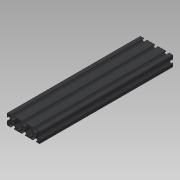
# Autodesk Inventor part: 1030
Saved by Autodesk Inventor 2013 (Build 170138000, 138)
## iProperties
Company: 80/20 Inc.
Created: 2013-09-06
Part Number: 1030
Material: Generic
Document SubType Name: Modeling
Density: 1 g/cm^3
Catalog Web Link: 8020.net
Vendor: 80/20 Inc.
Engineer: Ross Bowman
Author: Ross Bowman
Keywords: T-Slot, Extrusion, 80/20, 8020, Quick Frame, HT
Autodesk Inventor part; units mm, degrees
ref_plane "YZ Plane" through (0, 0, 0) normal (1, 0, 0) x (0, 1, 0)
ref_plane "XZ Plane" through (0, 0, 0) normal (0, 1, 0) x (-1, 0, 0)
ref_plane "XY Plane" through (0, 0, 0) normal (0, 0, 1) x (1, 0, 0)
sketch "Sketch1" plane through (0, 0, 0) normal (0, 0, 1) x (1, 0, 0)
  circle A0 centre (25.4, 0) radius 2.6035
  circle A1 centre (0, 0) radius 2.6035
  circle A2 centre (-25.4, 0) radius 2.6035
  arc A3 (19.9657, -3.8718) -> (20.8956, -1.6267) centre (17.7206, -1.6267) ccw
  line L0 (14.2657, -9.5718) -> (19.9657, -3.8718)
  arc A4 (13.1521, -10.033) -> (14.2657, -9.5718) centre (13.1521, -8.4582) ccw
  line L1 (12.2479, -10.033) -> (13.1521, -10.033)
  arc A5 (11.1343, -9.5718) -> (12.2479, -10.033) centre (12.2479, -8.4582) ccw
  line L2 (5.4343, -3.8717) -> (11.1343, -9.5718)
  arc A6 (4.5044, -1.6267) -> (5.4343, -3.8717) centre (7.6794, -1.6267) ccw
  line L3 (4.5044, 1.6267) -> (4.5044, -1.6267)
  arc A7 (5.4343, 3.8717) -> (4.5044, 1.6267) centre (7.6794, 1.6267) ccw
  line L4 (11.1343, 9.5718) -> (5.4343, 3.8717)
  arc A8 (12.2479, 10.033) -> (11.1343, 9.5718) centre (12.2479, 8.4582) ccw
  line L5 (13.1521, 10.033) -> (12.2479, 10.033)
  arc A9 (14.2657, 9.5718) -> (13.1521, 10.033) centre (13.1521, 8.4582) ccw
  line L6 (19.9657, 3.8717) -> (14.2657, 9.5718)
  arc A10 (20.8956, 1.6267) -> (19.9657, 3.8717) centre (17.7206, 1.6267) ccw
  line L7 (20.8956, -1.6267) -> (20.8956, 1.6267)
  arc A11 (-20.8956, -1.6267) -> (-19.9657, -3.8717) centre (-17.7206, -1.6267) ccw
  line L8 (-20.8956, 1.6267) -> (-20.8956, -1.6267)
  arc A12 (-19.9657, 3.8717) -> (-20.8956, 1.6267) centre (-17.7206, 1.6267) ccw
  line L9 (-14.2657, 9.5718) -> (-19.9657, 3.8717)
  arc A13 (-13.1521, 10.033) -> (-14.2657, 9.5718) centre (-13.1521, 8.4582) ccw
  line L10 (-12.2479, 10.033) -> (-13.1521, 10.033)
  arc A14 (-11.1343, 9.5718) -> (-12.2479, 10.033) centre (-12.2479, 8.4582) ccw
  line L11 (-5.4343, 3.8717) -> (-11.1343, 9.5718)
  arc A15 (-4.5044, 1.6267) -> (-5.4343, 3.8717) centre (-7.6794, 1.6267) ccw
  line L12 (-4.5044, -1.6267) -> (-4.5044, 1.6267)
  arc A16 (-5.4343, -3.8718) -> (-4.5044, -1.6267) centre (-7.6794, -1.6267) ccw
  line L13 (-11.1343, -9.5718) -> (-5.4343, -3.8718)
  arc A17 (-12.2479, -10.033) -> (-11.1343, -9.5718) centre (-12.2479, -8.4582) ccw
  line L14 (-13.1521, -10.033) -> (-12.2479, -10.033)
  arc A18 (-14.2657, -9.5718) -> (-13.1521, -10.033) centre (-13.1521, -8.4582) ccw
  line L15 (-19.9657, -3.8717) -> (-14.2657, -9.5718)
  arc A19 (-1.6267, -4.5044) -> (-3.8717, -5.4343) centre (-1.6267, -7.6794) ccw
  line L16 (-1.6267, -4.5044) -> (1.6267, -4.5044)
  arc A20 (3.8717, -5.4343) -> (1.6267, -4.5044) centre (1.6267, -7.6794) ccw
  line L17 (3.8717, -5.4343) -> (7.1932, -8.7558)
  arc A21 (6.4748, -10.4902) -> (7.1932, -8.7558) centre (6.4748, -9.4742) ccw
  line L18 (6.4748, -10.4902) -> (4.3561, -10.4902)
  arc A22 (4.3561, -10.4902) -> (4.3561, -12.7) centre (4.3561, -11.5951) ccw
  line L19 (4.3561, -12.7) -> (5.3086, -12.7)
  arc A23 (6.3246, -12.7) -> (5.3086, -12.7) centre (5.8166, -12.7) ccw
  line L20 (6.3246, -12.7) -> (9.5504, -12.7)
  arc A24 (10.5664, -12.7) -> (9.5504, -12.7) centre (10.0584, -12.7) ccw
  line L21 (10.5664, -12.7) -> (14.8336, -12.7)
  arc A25 (15.8496, -12.7) -> (14.8336, -12.7) centre (15.3416, -12.7) ccw
  line L22 (15.8496, -12.7) -> (19.0754, -12.7)
  arc A26 (20.0914, -12.7) -> (19.0754, -12.7) centre (19.5834, -12.7) ccw
  line L23 (20.0914, -12.7) -> (21.0439, -12.7)
  arc A27 (21.0439, -12.7) -> (21.0439, -10.4902) centre (21.0439, -11.5951) ccw
  line L24 (21.0439, -10.4902) -> (18.9252, -10.4902)
  arc A28 (18.2068, -8.7558) -> (18.9252, -10.4902) centre (18.9252, -9.4742) ccw
  line L25 (18.2068, -8.7558) -> (21.5283, -5.4343)
  arc A29 (23.7733, -4.5044) -> (21.5283, -5.4343) centre (23.7733, -7.6794) ccw
  line L26 (23.7733, -4.5044) -> (27.0267, -4.5044)
  arc A30 (29.2718, -5.4343) -> (27.0267, -4.5044) centre (27.0267, -7.6794) ccw
  line L27 (29.2718, -5.4343) -> (32.5932, -8.7558)
  arc A31 (31.8748, -10.4902) -> (32.5932, -8.7558) centre (31.8748, -9.4742) ccw
  line L28 (31.8748, -10.4902) -> (29.7561, -10.4902)
  arc A32 (29.7561, -10.4902) -> (29.7561, -12.7) centre (29.7561, -11.5951) ccw
  line L29 (29.7561, -12.7) -> (30.7086, -12.7)
  arc A33 (31.7246, -12.7) -> (30.7086, -12.7) centre (31.2166, -12.7) ccw
  line L30 (31.7246, -12.7) -> (34.9504, -12.7)
  arc A34 (35.9664, -12.7) -> (34.9504, -12.7) centre (35.4584, -12.7) ccw
  line L31 (35.9664, -12.7) -> (35.9918, -12.7)
  arc A35 (35.9918, -12.7) -> (38.1, -10.5918) centre (35.9918, -10.5918) ccw
  line L32 (38.1, -10.5918) -> (38.1, -10.5664)
  arc A36 (38.1, -9.5504) -> (38.1, -10.5664) centre (38.1, -10.0584) ccw
  line L33 (38.1, -9.5504) -> (38.1, -6.3246)
  arc A37 (38.1, -5.3086) -> (38.1, -6.3246) centre (38.1, -5.8166) ccw
  line L34 (38.1, -5.3086) -> (38.1, -4.3561)
  arc A38 (38.1, -4.3561) -> (35.8902, -4.3561) centre (36.9951, -4.3561) ccw
  line L35 (35.8902, -4.3561) -> (35.8902, -6.4748)
  arc A39 (34.1558, -7.1932) -> (35.8902, -6.4748) centre (34.8742, -6.4748) ccw
  line L36 (34.1558, -7.1932) -> (30.8343, -3.8717)
  arc A40 (29.9044, -1.6267) -> (30.8343, -3.8717) centre (33.0794, -1.6267) ccw
  line L37 (29.9044, -1.6267) -> (29.9044, 1.6267)
  arc A41 (30.8343, 3.8718) -> (29.9044, 1.6267) centre (33.0794, 1.6267) ccw
  line L38 (30.8343, 3.8718) -> (34.1558, 7.1932)
  arc A42 (35.8902, 6.4748) -> (34.1558, 7.1932) centre (34.8742, 6.4748) ccw
  line L39 (35.8902, 6.4748) -> (35.8902, 4.3561)
  arc A43 (35.8902, 4.3561) -> (38.1, 4.3561) centre (36.9951, 4.3561) ccw
  line L40 (38.1, 4.3561) -> (38.1, 5.3086)
  arc A44 (38.1, 6.3246) -> (38.1, 5.3086) centre (38.1, 5.8166) ccw
  line L41 (38.1, 6.3246) -> (38.1, 9.5504)
  arc A45 (38.1, 10.5664) -> (38.1, 9.5504) centre (38.1, 10.0584) ccw
  line L42 (38.1, 10.5664) -> (38.1, 10.5918)
  arc A46 (38.1, 10.5918) -> (35.9918, 12.7) centre (35.9918, 10.5918) ccw
  line L43 (35.9918, 12.7) -> (35.9664, 12.7)
  arc A47 (34.9504, 12.7) -> (35.9664, 12.7) centre (35.4584, 12.7) ccw
  line L44 (34.9504, 12.7) -> (31.7246, 12.7)
  arc A48 (30.7086, 12.7) -> (31.7246, 12.7) centre (31.2166, 12.7) ccw
  line L45 (30.7086, 12.7) -> (29.7561, 12.7)
  arc A49 (29.7561, 12.7) -> (29.7561, 10.4902) centre (29.7561, 11.5951) ccw
  line L46 (29.7561, 10.4902) -> (31.8748, 10.4902)
  arc A50 (32.5932, 8.7558) -> (31.8748, 10.4902) centre (31.8748, 9.4742) ccw
  line L47 (32.5932, 8.7558) -> (29.2717, 5.4343)
  arc A51 (27.0267, 4.5044) -> (29.2717, 5.4343) centre (27.0267, 7.6794) ccw
  line L48 (27.0267, 4.5044) -> (23.7733, 4.5044)
  arc A52 (21.5283, 5.4343) -> (23.7733, 4.5044) centre (23.7733, 7.6794) ccw
  line L49 (21.5283, 5.4343) -> (18.2068, 8.7558)
  arc A53 (18.9252, 10.4902) -> (18.2068, 8.7558) centre (18.9252, 9.4742) ccw
  line L50 (18.9252, 10.4902) -> (21.0439, 10.4902)
  arc A54 (21.0439, 10.4902) -> (21.0439, 12.7) centre (21.0439, 11.5951) ccw
  line L51 (21.0439, 12.7) -> (20.0914, 12.7)
  arc A55 (19.0754, 12.7) -> (20.0914, 12.7) centre (19.5834, 12.7) ccw
  line L52 (19.0754, 12.7) -> (15.8496, 12.7)
  arc A56 (14.8336, 12.7) -> (15.8496, 12.7) centre (15.3416, 12.7) ccw
  line L53 (14.8336, 12.7) -> (10.5664, 12.7)
  arc A57 (9.5504, 12.7) -> (10.5664, 12.7) centre (10.0584, 12.7) ccw
  line L54 (9.5504, 12.7) -> (6.3246, 12.7)
  arc A58 (5.3086, 12.7) -> (6.3246, 12.7) centre (5.8166, 12.7) ccw
  line L55 (5.3086, 12.7) -> (4.3561, 12.7)
  arc A59 (4.3561, 12.7) -> (4.3561, 10.4902) centre (4.3561, 11.5951) ccw
  line L56 (4.3561, 10.4902) -> (6.4748, 10.4902)
  arc A60 (7.1932, 8.7558) -> (6.4748, 10.4902) centre (6.4748, 9.4742) ccw
  line L57 (7.1932, 8.7558) -> (3.8717, 5.4343)
  arc A61 (1.6267, 4.5044) -> (3.8717, 5.4343) centre (1.6267, 7.6794) ccw
  line L58 (1.6267, 4.5044) -> (-1.6267, 4.5044)
  arc A62 (-3.8717, 5.4343) -> (-1.6267, 4.5044) centre (-1.6267, 7.6794) ccw
  line L59 (-3.8717, 5.4343) -> (-7.1932, 8.7558)
  arc A63 (-6.4748, 10.4902) -> (-7.1932, 8.7558) centre (-6.4748, 9.4742) ccw
  line L60 (-6.4748, 10.4902) -> (-4.3561, 10.4902)
  arc A64 (-4.3561, 10.4902) -> (-4.3561, 12.7) centre (-4.3561, 11.5951) ccw
  line L61 (-4.3561, 12.7) -> (-5.3086, 12.7)
  arc A65 (-6.3246, 12.7) -> (-5.3086, 12.7) centre (-5.8166, 12.7) ccw
  line L62 (-6.3246, 12.7) -> (-9.5504, 12.7)
  arc A66 (-10.5664, 12.7) -> (-9.5504, 12.7) centre (-10.0584, 12.7) ccw
  line L63 (-10.5664, 12.7) -> (-14.8336, 12.7)
  arc A67 (-15.8496, 12.7) -> (-14.8336, 12.7) centre (-15.3416, 12.7) ccw
  line L64 (-15.8496, 12.7) -> (-19.0754, 12.7)
  arc A68 (-20.0914, 12.7) -> (-19.0754, 12.7) centre (-19.5834, 12.7) ccw
  line L65 (-20.0914, 12.7) -> (-21.0414, 12.7)
  arc A69 (-21.0414, 12.7) -> (-21.0414, 10.4902) centre (-21.0414, 11.5951) ccw
  line L66 (-21.0414, 10.4902) -> (-18.9252, 10.4902)
  arc A70 (-18.2068, 8.7558) -> (-18.9252, 10.4902) centre (-18.9252, 9.4742) ccw
  line L67 (-18.2068, 8.7558) -> (-21.5283, 5.4343)
  arc A71 (-23.7733, 4.5044) -> (-21.5283, 5.4343) centre (-23.7733, 7.6794) ccw
  line L68 (-23.7733, 4.5044) -> (-27.0267, 4.5044)
  arc A72 (-29.2717, 5.4343) -> (-27.0267, 4.5044) centre (-27.0267, 7.6794) ccw
  line L69 (-29.2717, 5.4343) -> (-32.5932, 8.7558)
  arc A73 (-31.8748, 10.4902) -> (-32.5932, 8.7558) centre (-31.8748, 9.4742) ccw
  line L70 (-31.8748, 10.4902) -> (-29.7561, 10.4902)
  arc A74 (-29.7561, 10.4902) -> (-29.7561, 12.7) centre (-29.7561, 11.5951) ccw
  line L71 (-29.7561, 12.7) -> (-30.7086, 12.7)
  arc A75 (-31.7246, 12.7) -> (-30.7086, 12.7) centre (-31.2166, 12.7) ccw
  line L72 (-31.7246, 12.7) -> (-34.9504, 12.7)
  arc A76 (-35.9664, 12.7) -> (-34.9504, 12.7) centre (-35.4584, 12.7) ccw
  line L73 (-35.9664, 12.7) -> (-35.9918, 12.7)
  arc A77 (-35.9918, 12.7) -> (-38.1, 10.5918) centre (-35.9918, 10.5918) ccw
  line L74 (-38.1, 10.5918) -> (-38.1, 10.5664)
  arc A78 (-38.1, 9.5504) -> (-38.1, 10.5664) centre (-38.1, 10.0584) ccw
  line L75 (-38.1, 9.5504) -> (-38.1, 6.3246)
  arc A79 (-38.1, 5.3086) -> (-38.1, 6.3246) centre (-38.1, 5.8166) ccw
  line L76 (-38.1, 5.3086) -> (-38.1, 4.3561)
  arc A80 (-38.1, 4.3561) -> (-35.8902, 4.3561) centre (-36.9951, 4.3561) ccw
  line L77 (-35.8902, 4.3561) -> (-35.8902, 6.4748)
  arc A81 (-34.1558, 7.1932) -> (-35.8902, 6.4748) centre (-34.8742, 6.4748) ccw
  line L78 (-34.1558, 7.1932) -> (-30.8343, 3.8717)
  arc A82 (-29.9044, 1.6267) -> (-30.8343, 3.8717) centre (-33.0794, 1.6267) ccw
  line L79 (-29.9044, 1.6267) -> (-29.9044, -1.6267)
  arc A83 (-30.8343, -3.8717) -> (-29.9044, -1.6267) centre (-33.0794, -1.6267) ccw
  line L80 (-30.8343, -3.8717) -> (-34.1558, -7.1932)
  arc A84 (-35.8902, -6.4748) -> (-34.1558, -7.1932) centre (-34.8742, -6.4748) ccw
  line L81 (-35.8902, -6.4748) -> (-35.8902, -4.3561)
  arc A85 (-35.8902, -4.3561) -> (-38.1, -4.3561) centre (-36.9951, -4.3561) ccw
  line L82 (-38.1, -4.3561) -> (-38.1, -5.3086)
  arc A86 (-38.1, -6.3246) -> (-38.1, -5.3086) centre (-38.1, -5.8166) ccw
  line L83 (-38.1, -6.3246) -> (-38.1, -9.5504)
  arc A87 (-38.1, -10.5664) -> (-38.1, -9.5504) centre (-38.1, -10.0584) ccw
  line L84 (-38.1, -10.5664) -> (-38.1, -10.5918)
  arc A88 (-38.1, -10.5918) -> (-35.9918, -12.7) centre (-35.9918, -10.5918) ccw
  line L85 (-35.9918, -12.7) -> (-35.9664, -12.7)
  arc A89 (-34.9504, -12.7) -> (-35.9664, -12.7) centre (-35.4584, -12.7) ccw
  line L86 (-34.9504, -12.7) -> (-31.7246, -12.7)
  arc A90 (-30.7086, -12.7) -> (-31.7246, -12.7) centre (-31.2166, -12.7) ccw
  line L87 (-30.7086, -12.7) -> (-29.7561, -12.7)
  arc A91 (-29.7561, -12.7) -> (-29.7561, -10.4902) centre (-29.7561, -11.5951) ccw
  line L88 (-29.7561, -10.4902) -> (-31.8748, -10.4902)
  arc A92 (-32.5932, -8.7558) -> (-31.8748, -10.4902) centre (-31.8748, -9.4742) ccw
  line L89 (-32.5932, -8.7558) -> (-29.2717, -5.4343)
  arc A93 (-27.0267, -4.5044) -> (-29.2717, -5.4343) centre (-27.0267, -7.6794) ccw
  line L90 (-27.0267, -4.5044) -> (-23.7733, -4.5044)
  arc A94 (-21.5283, -5.4343) -> (-23.7733, -4.5044) centre (-23.7733, -7.6794) ccw
  line L91 (-21.5283, -5.4343) -> (-18.2068, -8.7558)
  arc A95 (-18.9252, -10.4902) -> (-18.2068, -8.7558) centre (-18.9252, -9.4742) ccw
  line L92 (-18.9252, -10.4902) -> (-21.0414, -10.4902)
  arc A96 (-21.0414, -10.4902) -> (-21.0414, -12.7) centre (-21.0414, -11.5951) ccw
  line L93 (-21.0414, -12.7) -> (-20.0914, -12.7)
  arc A97 (-19.0754, -12.7) -> (-20.0914, -12.7) centre (-19.5834, -12.7) ccw
  line L94 (-19.0754, -12.7) -> (-15.8496, -12.7)
  arc A98 (-14.8336, -12.7) -> (-15.8496, -12.7) centre (-15.3416, -12.7) ccw
  line L95 (-14.8336, -12.7) -> (-10.5664, -12.7)
  arc A99 (-9.5504, -12.7) -> (-10.5664, -12.7) centre (-10.0584, -12.7) ccw
  line L96 (-9.5504, -12.7) -> (-6.3246, -12.7)
  arc A100 (-5.3086, -12.7) -> (-6.3246, -12.7) centre (-5.8166, -12.7) ccw
  line L97 (-5.3086, -12.7) -> (-4.3561, -12.7)
  arc A101 (-4.3561, -12.7) -> (-4.3561, -10.4902) centre (-4.3561, -11.5951) ccw
  line L98 (-4.3561, -10.4902) -> (-6.4748, -10.4902)
  arc A102 (-7.1932, -8.7558) -> (-6.4748, -10.4902) centre (-6.4748, -9.4742) ccw
  line L99 (-7.1932, -8.7558) -> (-3.8717, -5.4343)
  constraints: 200 end point, 200 point on circle, 103 centre point
extrude "Extrusion1" add sketch "Sketch1" against normal blind 304.8
body "Solid1"
